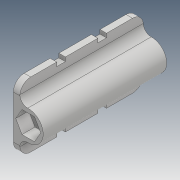
# Autodesk Inventor part: Soporte ESC
Saved by Autodesk Inventor 2017 (Build 210142000, 142)
## iProperties
Part Number: Soporte ESC
Material: Genérico
Document SubType Name: Modeling
Designer: beta3
Density: 1 g/cm^3
Appearance: Valor por defecto
Author: beta3
Autodesk Inventor part; units mm, degrees
ref_plane "YZ Plane" through (0, 0, 0) normal (1, 0, 0) x (0, 1, 0)
ref_plane "XZ Plane" through (0, 0, 0) normal (0, 1, 0) x (-1, 0, 0)
ref_plane "XY Plane" through (0, 0, 0) normal (0, 0, 1) x (1, 0, 0)
sketch "Boceto1" plane through (0, 0, 0) normal (0, 1, 0) x (-1, 0, 0)
  circle A0 centre (0, 0) radius 3.15
  line L0 (6.889, 15) -> (3.889, 15)
  line L1 (3.889, -15) -> (6.889, -15)
  line L2 (6.889, -15) -> (6.889, 15)
  line L3 (0, 0) -> (3.15, 0) construction
  arc A1 (0.2346, 6.885) -> (0.2346, -6.885) centre (0, 0) ccw
  line L4 (3.889, 15) -> (3.889, 10.4169)
  line L5 (3.889, -15) -> (3.889, -10.4169)
  arc A2 (0.2346, 6.885) -> (3.889, 10.4169) centre (0.355, 10.4169) ccw
  arc A3 (3.889, -10.4169) -> (0.2346, -6.885) centre (0.355, -10.4169) ccw
  line L6 (2.9445, 5.1) -> (5.889, 0) construction
  line L7 (5.889, 0) -> (2.9445, -5.1) construction
  line L8 (2.9445, -5.1) -> (-2.9445, -5.1) construction
  line L9 (-2.9445, -5.1) -> (-5.889, 0) construction
  line L10 (-5.889, 0) -> (-2.9445, 5.1) construction
  line L11 (-2.9445, 5.1) -> (2.9445, 5.1) construction
  line L12 (5.889, 0) -> (6.889, 0) construction
  line L13 (-5.889, 0) -> (-6.889, 0) construction
  dimension "d0" = 6.3
  dimension "d3" = 10.2
  dimension "d4" = 1
  dimension "d5" = 3
  dimension "d12" = 30
  constraints: 28 end point, 7 point on circle, 4 symmetric about line, 4 tangent, 3 centre point, 3 coincident, 3 horizontal, 2 vertical, 1 collinear, 1 horizontal alignment, 1 midpoint, 1 parallel, 15 other
  measures "d3" distance between parallel lines of L8 L11
  measures "d4" distance of L6.end L12.end
  measures "d5" distance of L1.start L1.end
  measures "d12" distance of L1.end L0.start
extrude "Extrusión1" add sketch "Boceto1" along normal blind 57
sketch "Boceto2" plane through (0, 0, 0) normal (0, -1, 0) x (1, 0, 0)
  line L0 (-5.7735, 0) -> (-2.8868, 5)
  line L1 (-2.8868, 5) -> (2.8868, 5)
  line L2 (2.8868, 5) -> (5.7735, 0)
  line L3 (5.7735, 0) -> (2.8868, -5)
  line L4 (2.8868, -5) -> (-2.8868, -5)
  line L5 (-2.8868, -5) -> (-5.7735, 0)
  point P0 (0, 0)
  point P1 (0, 0)
  dimension "d8" = 10
  constraints: 12 end point, 1 coincident, 13 other
  measures "d8" distance between parallel lines of L4 L1
extrude "Extrusión2" cut sketch "Boceto2" against normal blind 6
sketch "Boceto4" plane through (-6.889, 0, -15) normal (-1, 0, 0) x (0, 0, 1)
  line L0 (0, 0) -> (0, 57) projected
  line L1 (0, 28.5) -> (30, 28.5) construction
  line L2 (30, 0) -> (30, 57) projected
  line L3 (0, 36) -> (2, 36)
  line L4 (2, 36) -> (2, 40)
  line L5 (2, 40) -> (0, 40)
  line L6 (0, 40) -> (0, 36)
  line L7 (30, 36) -> (28.1744, 36)
  line L8 (28.1744, 36) -> (28.1744, 40)
  line L9 (28.1744, 40) -> (30, 40)
  line L10 (30, 40) -> (30, 36)
  line L11 (0, 21) -> (2, 21)
  line L12 (2, 21) -> (2, 17)
  line L13 (2, 17) -> (0, 17)
  line L14 (0, 17) -> (0, 21)
  line L15 (30, 21) -> (28.1744, 21)
  line L16 (28.1744, 21) -> (28.1744, 17)
  line L17 (28.1744, 17) -> (30, 17)
  line L18 (30, 17) -> (30, 21)
  line L19 (2, 40) -> (28.1744, 40) construction
  line L20 (2, 36) -> (28.1744, 36) construction
  line L21 (2, 21) -> (28.1744, 21) construction
  line L22 (2, 17) -> (28.1744, 17) construction
  point P0 (15, 0)
  dimension "d13" = 2
  dimension "d14" = 4
  dimension "d15" = 15
  constraints: 42 end point, 9 parallel, 8 horizontal, 7 point on line, 4 perpendicular, 2 midpoint, 2 symmetric about line
  measures "d13" distance of L4.end L5.end
  measures "d14" distance of L3.end L4.end
  measures "d15" distance between parallel lines of L21 L20
extrude "Extrusión3" cut sketch "Boceto4" against normal up to next
fillet "Empalme1" radius 5 4 edges at (-5.389, 57, -15) (-5.389, 57, 15) (-5.389, 0, 15) (-5.389, 0, -15)
